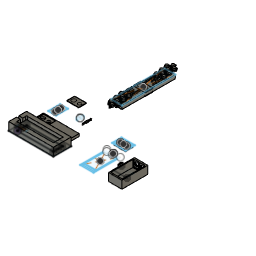
2020_09_27_9V Led 1W Experiments v4 (Autodesk Fusion 360 design; units mm, degrees)
Autodesk Fusion 360 part; units mm, degrees
sketch "Sketch1" plane through (0, 0, 0) normal (0, 0, 1) x (1, 0, 0)
  line L0 (0, 0) -> (80, 0)
  line L1 (80, 0) -> (80, 20)
  line L2 (80, 20) -> (0, 20)
  line L3 (0, 20) -> (0, 0)
  line L4 (-10, -10) -> (90, -10)
  line L5 (90, -10) -> (90, 30)
  line L6 (90, 30) -> (-10, 30)
  line L7 (-10, 30) -> (-10, -10)
  circle A0 centre (0, 20) radius 1.6
  circle A1 centre (80, 20) radius 1.6
  circle A2 centre (80, 0) radius 1.6
  circle A3 centre (0, 0) radius 1.6
  line L8 (-10, 12.5) -> (10, 12.5)
  line L9 (10, 12.5) -> (10, 7.5)
  line L10 (10, 7.5) -> (-10, 7.5)
  line L11 (-10, 7.5) -> (-10, 12.5)
  line L12 (-10, 12.5) -> (10, 7.5) construction
  line L13 (10, 12.5) -> (-10, 7.5) construction
  circle A4 centre (80, 10) radius 1.55
  line L14 (-1, -1) -> (81, -1)
  line L15 (81, -1) -> (81, 21)
  line L16 (81, 21) -> (-1, 21)
  line L17 (-1, 21) -> (-1, -1)
  point P0 (-10, 10)
  point P1 (0, 10)
  dimension "d1" = 80
  dimension "d2" = 20
  dimension "d3" = 10
  dimension "d10" = 3.2
  dimension "d12" = 5
  dimension "d18" = 3.1
  dimension "d21" = 1
  constraint horizontal L0
  constraint vertical L1
  constraint horizontal L2
  constraint vertical L3
  constraint coincident L0.start L3.end
  constraint coincident L2.end L3.start
  constraint coincident L1.end L2.start
  constraint coincident L0.end L1.start
  constraint equal A0 A1
  constraint equal A0 A3
  constraint equal A0 A2
  constraint midpoint L7 P0
  constraint horizontal L8
  constraint perpendicular L8 L9
  constraint parallel L8 L10
  constraint parallel L9 L11
  constraint coincident L12 P1
  constraint coincident L13 P1
  constraint midpoint L3 P1
  constraint midpoint L1 A4.centre
  measures "d1" distance of L0.start L0.end
  measures "d2" distance of L0.start L2.end
  measures "d10" diameter of A0
  measures "d12" distance of L8.end L9.end
  measures "d18" diameter of A4
extrude "Extrude1" add sketch "Sketch1" along normal blind 17.8 contours L4 L5 L6 L7 A0 A1 A2 A3 L8 L10 A4 L14 L15 L16 L17 makes body 1
extrude "Extrude3" add sketch "Sketch1" along normal blind 5.3 separate body contours L0 L3 A3 | L0 L3 A3 L14 L17 | L0 L1 L2 L3 A0 A1 A2 A3 L8 L9 L10 A4 | L0 A2 A3 L14 | L3 A3 L10 L17 | L0 L1 A2 | L0 L1 A2 L14 L15 | A3 L14 L17 | L3 L8 L10 L17 | L3 L8 L9 L10 | L1 A2 A4 L15 | A2 L14 L15 | L3 A0 L8 L17 | L1 A4 | L1 A4 L15 | L2 L3 A0 L16 L17 | L2 L3 A0 | L1 A1 A4 L15 | A4 L15 | A0 L16 L17 | L2 A0 A1 L16 | L1 L2 A1 | L1 L2 A1 L15 L16 | A1 L15 L16 makes body 2
move_body "Move1" bodies 2 to x (1, 0, 0) y (0, 1, 0) z (0, 0, 1) at (0, 0, 5.3)
extrude "Extrude4" add sketch "Sketch1" along normal blind 10.6 contours L0 L3 A3 | L0 L3 A3 L14 L17 | L0 L1 L2 L3 A0 A1 A2 A3 L8 L9 L10 A4 | L0 L1 A2 | L0 L1 A2 L14 L15 | A3 L14 L17 | A2 L14 L15 | L1 A4 | L1 A4 L15 | L2 L3 A0 L16 L17 | L2 L3 A0 | A4 L15 | A0 L16 L17 | L1 L2 A1 | L1 L2 A1 L15 L16 | A1 L15 L16 bodies 2 1
extrude "Extrude5" add sketch "Sketch1" along normal blind 5.5 separate body contours L0 L3 A3 | L0 L1 L2 L3 A0 A1 A2 A3 L8 L9 L10 A4 | L0 L1 A2 | L3 L8 L9 L10 | L1 A4 | L2 L3 A0 | L1 L2 A1 makes body 3
move_body "Move2" bodies 3 to x (1, 0, 0) y (0, 1, 0) z (0, 0, 1) at (0, 38, 0)
sketch "Sketch2" plane through (0, 0, 0) normal (1, 0, 0) x (0, 1, 0)
sketch "SquareBattery" plane through (0, 0, 0) normal (0, 0, 1) x (1, 0, 0)
  circle A0 centre (4.7694, 92.4101) radius 3.5
  circle A1 centre (4.7694, 79.4101) radius 4.5
  line L0 (4.7694, 79.4101) -> (4.7694, 92.4101)
  line L1 (13.5194, 99.1601) -> (-3.9806, 99.1601)
  line L2 (-3.9806, 99.1601) -> (-3.9806, 72.6601)
  line L3 (-3.9806, 72.6601) -> (13.5194, 72.6601)
  line L4 (13.5194, 72.6601) -> (13.5194, 99.1601)
  line L5 (13.5194, 99.1601) -> (-3.9806, 72.6601) construction
  line L6 (-3.9806, 99.1601) -> (13.5194, 72.6601) construction
  point P0 (4.7694, 85.9101)
  point P1 (4.7694, 85.9101)
  dimension "d25" = 7
  dimension "d26" = 9
  dimension "d27" = 13
  dimension "d28" = 17.5
  dimension "d29" = 26.5
  constraint coincident A1.centre L0.start
  constraint vertical L0
  constraint coincident A0.centre L0.end
  constraint midpoint L0 P1
  constraint horizontal L1
  constraint perpendicular L1 L2
  constraint parallel L1 L3
  constraint parallel L2 L4
  constraint coincident L5 P1
  constraint coincident L6 P1
  constraint coincident P1 P0
  measures "d25" diameter of A0
  measures "d26" diameter of A1
  measures "d27" distance of A1.centre A0.centre
  measures "d28" distance of L2.end L3.end
  measures "d29" distance of L1.end L2.end
extrude "Extrude6" add sketch "SquareBattery" against normal blind 3 separate body contours A0 | A1 makes body 4 at (8.0583, 91.2131, -2) makes body 5 at (9.247, 79.8582, -1)
extrude "Extrude7" add sketch "SquareBattery" along normal blind 1 contours A0 | A1 | L1 L2 L3 L4 bodies 4 5
move_body "Move3" bodies 4 to x (0, -1, 0) y (1, 0, 0) z (0, 0, 1) at (-58, 58, 0)
move_body "Move4" bodies 4 to x (1, 0, 0) y (0, 1, 0) z (0, 0, 1) at (-14.6601, -5.2306, 4.5)
move_body "Move5" bodies 4 to x (1, 0, 0) y (0, 1, 0) z (0, 0, 1) at (2, 0, 0)
copy_body "CopyPasteBodies1" bodies 4 makes body 6
move_body "Move6" bodies 6 to x (1, 0, 0) y (0, 1, 0) z (0, 0, 1) at (0, 69, 0)
combine "Combine1" operation cut target body 3 tool bodies 4
sketch "Zerodis6bz7yhokr1-02" plane through (0, 0, 0) normal (0, 0, 1) x (1, 0, 0)
  line L0 (41.1745, 98.5288) -> (49.3245, 98.5288)
  line L1 (49.3245, 98.5288) -> (49.3245, 91.2088)
  line L2 (49.3245, 91.2088) -> (41.1745, 91.2088)
  line L3 (41.1745, 91.2088) -> (41.1745, 98.5288)
  line L4 (45.2495, 98.5288) -> (45.2495, 91.2088) construction
  arc A0 (43.4578, 98.5288) -> (43.4578, 91.2088) centre (45.2495, 94.8688) ccw
  arc A1 (47.0411, 91.2088) -> (47.0411, 98.5288) centre (45.2495, 94.8688) ccw
  circle A2 centre (45.2495, 94.8688) radius 2.75
  line L5 (45.2495, 98.5288) -> (43.4578, 98.5288)
  line L6 (43.4578, 98.5288) -> (43.4578, 102.2288)
  line L7 (43.4578, 102.2288) -> (45.2495, 102.2288)
  line L8 (45.2495, 102.2288) -> (45.2495, 98.5288)
  line L9 (45.2495, 91.2088) -> (47.0411, 91.2088)
  line L10 (47.0411, 91.2088) -> (47.0411, 87.5088)
  line L11 (47.0411, 87.5088) -> (45.2495, 87.5088)
  line L12 (45.2495, 87.5088) -> (45.2495, 91.2088)
  line L13 (45.2495, 98.5288) -> (45.2495, 100.5288)
  line L14 (45.2495, 100.5288) -> (43.4578, 100.5288)
  line L15 (45.2495, 91.2088) -> (45.2495, 89.2088)
  line L16 (45.2495, 89.2088) -> (47.0411, 89.2088)
  line L17 (47.0411, 98.5288) -> (45.2495, 98.5288)
  line L18 (45.2495, 98.5288) -> (45.2495, 100.0288)
  line L19 (45.2495, 100.0288) -> (47.0411, 100.0288)
  line L20 (47.0411, 100.0288) -> (47.0411, 98.5288)
  line L21 (43.4578, 91.2088) -> (45.2495, 91.2088)
  line L22 (45.2495, 91.2088) -> (45.2495, 89.7088)
  line L23 (45.2495, 89.7088) -> (43.4578, 89.7088)
  line L24 (43.4578, 89.7088) -> (43.4578, 91.2088)
  dimension "d38" = 8.15
  dimension "d39" = 7.32
  dimension "d42" = 5.5
  dimension "d43" = 3.7
  dimension "d44" = 3.7
  dimension "d51" = 2
  dimension "d52" = 2
  dimension "d55" = 1.5
  dimension "d56" = 1.5
  constraint horizontal L0
  constraint vertical L1
  constraint horizontal L2
  constraint vertical L3
  constraint midpoint L0 L4.start
  constraint midpoint L2 L4.end
  constraint tangent L1 A0
  constraint coincident L0 A1.end
  constraint coincident L0 A0.start
  constraint coincident L2 A0.end
  constraint coincident L2 A1.start
  constraint concentric A0 A1
  constraint horizontal L5
  constraint vertical L6
  constraint horizontal L7
  constraint vertical L8
  constraint horizontal L9
  constraint vertical L10
  constraint horizontal L11
  constraint vertical L12
  constraint perpendicular L0 L13
  constraint coincident L6 L14.end
  constraint perpendicular L6 L14
  constraint perpendicular L2 L15
  constraint coincident L10 L16.end
  constraint perpendicular L10 L16
  constraint horizontal L17
  constraint vertical L18
  constraint horizontal L19
  constraint vertical L20
  constraint horizontal L21
  constraint vertical L22
  constraint horizontal L23
  constraint vertical L24
  measures "d38" distance of L0.start L0.end
  measures "d39" distance of L0.start L2.end
  measures "d42" diameter of A2
  measures "d43" distance of L4.start L7.end
  measures "d44" distance of L4.end L11.end
  measures "d51" distance of L4.start L13.end
  measures "d52" distance of L4.end L15.end
  measures "d55" distance of A1.end L19.end
  measures "d56" distance of A0.end L23.end
extrude "Extrude8" add sketch "Zerodis6bz7yhokr1-02" against normal blind 0.1 separate body contours L0 L5 L6 L8 L13 L14 L18 | L6 L7 L8 L14 | L2 L9 L10 L12 L15 L16 L22 | L10 L11 L12 L16 makes body 7 at (46.4439, 89.9755, 0) makes body 8 at (44.055, 100.9955, 0)
extrude "Extrude9" add sketch "Zerodis6bz7yhokr1-02" along normal blind 2.37 separate body contours L0 L2 A0 A1 L5 L9 L17 L21 | A2 makes body 9
extrude "Extrude10" add sketch "Zerodis6bz7yhokr1-02" along normal blind 5.1 contours A2 bodies 9
extrude "Extrude11" add sketch "Zerodis6bz7yhokr1-02" along normal blind 1.8 contours L0 L5 L6 L8 L13 L14 L18 | L2 L9 L10 L12 L15 L16 L22 bodies 7 8 9
extrude "Extrude12" add sketch "Zerodis6bz7yhokr1-02" along normal blind 1.8 contours L0 L8 L13 L17 L18 L19 L20 | L2 L12 L15 L21 L22 L23 L24 bodies 7
extrude "Extrude13" add sketch "Zerodis6bz7yhokr1-02" along normal blind 0.15 contours L6 L7 L8 L14 | L10 L11 L12 L16 bodies 7
copy_body "CopyPasteBodies2" bodies 7 makes body 10
move_body "Move7" bodies 10 to x (1, 0, 0) y (0, 1, 0) z (0, 0, 1) at (0, 200, 0)
copy_body "CopyPasteBodies3" bodies 10 makes body 11
move_body "Move8" bodies 11 to x (1, 0, 0) y (0, 1, 0) z (0, 0, 1) at (1.8025, -13.4584, 0)
copy_body "CopyPasteBodies4" bodies 11 makes body 12
move_body "Move9" bodies 12 to x (1, 0, 0) y (0, 1, 0) z (0, 0, 1) at (1.8025, -13.3382, 0)
copy_body "CopyPasteBodies5" bodies 10 12 11 makes body 13 makes body 14 makes body 15
move_body "Move10" bodies 13 14 15 to x (1, 0, 0) y (0, 1, 0) z (0, 0, 1) at (5.2658, 8.138, 0)
copy_body "CopyPasteBodies6" bodies 13 14 15 makes body 16 makes body 17 makes body 18
move_body "Move11" bodies 16 17 18 to x (1, 0, 0) y (0, 1, 0) z (0, 0, 1) at (7.5995, -5.0264, 0)
move_body "Move12" bodies 10 12 11 to x (1, 0, 0) y (0, 1, 0) z (0, 0, 1) at (-1, 0, 0)
sketch "Resistance" plane through (0, 0, 0) normal (0, 0, 1) x (1, 0, 0)
  line L0 (60.0185, 97.4679) -> (62.6185, 97.4679)
  line L1 (62.6185, 97.4679) -> (62.6185, 90.0679)
  line L2 (62.6185, 90.0679) -> (60.0185, 90.0679)
  line L3 (60.0185, 90.0679) -> (60.0185, 97.4679)
  line L4 (60.0185, 93.7679) -> (62.6185, 93.7679) construction
  line L5 (61.8685, 102.8813) -> (60.7685, 102.8813)
  line L6 (60.7685, 102.8813) -> (60.7685, 84.6546)
  line L7 (60.7685, 84.6546) -> (61.8685, 84.6546)
  line L8 (61.8685, 84.6546) -> (61.8685, 102.8813)
  line L9 (61.8685, 102.8813) -> (60.7685, 84.6546) construction
  line L10 (60.7685, 102.8813) -> (61.8685, 84.6546) construction
  circle A0 centre (61.3185, 84.6546) radius 1.25
  circle A1 centre (61.3185, 102.8813) radius 1.25
  point P0 (61.3185, 93.7679)
  dimension "d64" = 2.6
  dimension "d65" = 7.4
  dimension "d66" = 1.1
  dimension "d67" = 2.5
  dimension "d68" = 2.5
  constraint horizontal L0
  constraint vertical L1
  constraint horizontal L2
  constraint vertical L3
  constraint midpoint L3 L4.start
  constraint midpoint L1 L4.end
  constraint horizontal L5
  constraint perpendicular L5 L6
  constraint parallel L5 L7
  constraint parallel L6 L8
  constraint coincident L9 P0
  constraint coincident L10 P0
  constraint midpoint L4 P0
  constraint midpoint L7 A0.centre
  constraint midpoint L5 A1.centre
  measures "d64" distance of L0.start L0.end
  measures "d65" distance of L0.start L2.end
  measures "d66" distance of L6.end L7.end
  measures "d67" diameter of A0
  measures "d68" diameter of A1
extrude "Extrude14" add sketch "Resistance" along normal blind 2.5 separate body makes body 19
copy_body "CopyPasteBodies7" bodies 19 makes body 20
move_body "Move13" bodies 20 to x (1, 0, 0) y (0, 1, 0) z (0, 0, 1) at (1.3709, 160.9305, 0)
copy_body "CopyPasteBodies8" bodies 20 makes body 21
move_body "Move14" bodies 21 to x (1, 0, 0) y (0, 1, 0) z (0, 0, 1) at (-7.5014, 5.0154, 0)
copy_body "CopyPasteBodies9" bodies 21 makes body 22
move_body "Move15" bodies 22 to x (1, 0, 0) y (0, 1, 0) z (0, 0, 1) at (-6.3238, -7.9811, 0)
copy_body "CopyPasteBodies10" bodies 6 makes body 23
move_body "Move16" bodies 23 to x (1, 0, 0) y (0, 1, 0) z (0, 0, 1) at (39.8975, 108.9439, 0)
copy_body "CopyPasteBodies11" bodies 10 12 11 13 14 15 18 17 16 20 21 22 makes body 24 makes body 25 makes body 26 makes body 27 makes body 28 makes body 29 makes body 30 makes body 31 makes body 32 makes body 33 makes body 34 makes body 35
move_body "Move17" bodies 24 25 26 27 28 29 30 31 32 33 34 35 to x (-1, 0, 0) y (0, -1, 0) z (0, 0, 1) at (123.2951, 451.8879, 0)
move_body "Move18" bodies 26 35 32 28 27 24 25 33 34 29 30 31 to x (1, 0, 0) y (0, 1, 0) z (0, 0, 1) at (-15, 5, 0)
move_body "Move19" bodies 15 17 12 22 10 13 21 11 20 18 14 16 to x (1, 0, 0) y (0, 1, 0) z (0, 0, 1) at (0, -5, 0)
sketch "Sketch6" plane through (0, 0, 0) normal (0, 0, 1) x (1, 0, 0)
  line L0 (67.6833, 285.9439) -> (43.6833, 285.9439)
  line L1 (43.6833, 285.9439) -> (43.6833, 165.9439)
  line L2 (43.6833, 165.9439) -> (67.6833, 165.9439)
  line L3 (67.6833, 165.9439) -> (67.6833, 285.9439)
  line L4 (67.6833, 285.9439) -> (43.6833, 165.9439) construction
  line L5 (43.6833, 285.9439) -> (67.6833, 165.9439) construction
  point P0 (55.6833, 225.9439)
  dimension "d78" = 24
  dimension "d79" = 120
  constraint horizontal L0
  constraint perpendicular L0 L1
  constraint parallel L0 L2
  constraint parallel L1 L3
  constraint coincident L4 P0
  constraint coincident L5 P0
  measures "d78" distance of L1.end L2.end
  measures "d79" distance of L0.end L1.end
extrude "Extrude15" add sketch "Sketch6" against normal blind 8 separate body makes body 36
move_body "Move20" bodies 23 to x (1, 0, 0) y (0, 1, 0) z (0, 0, 1) at (0, 0, -5.5)
copy_body "CopyPasteBodies12" bodies 23 makes body 37
move_body "Move21" bodies 37 to x (-1, 0, 0) y (0, 1, 0) z (0, 0, -1) at (83.7951, 0, 0)
move_body "Move22" bodies 37 to x (1, 0, 0) y (0, 1, 0) z (0, 0, 1) at (26.5, 0, -8)
sketch "Sketch7" plane through (0, 0, 0) normal (0, 0, 1) x (1, 0, 0)
  line L0 (138.4181, 56.7453) -> (164.4181, 56.7453)
  line L1 (164.4181, 56.7453) -> (164.4181, 10.7453)
  line L2 (164.4181, 10.7453) -> (138.4181, 10.7453)
  line L3 (138.4181, 10.7453) -> (138.4181, 56.7453)
  line L4 (138.4181, 33.7453) -> (164.4181, 33.7453) construction
  line L5 (136.4181, 61.2453) -> (136.4181, 3.7453)
  line L6 (136.4181, 3.7453) -> (166.4181, 3.7453)
  line L7 (166.4181, 3.7453) -> (166.4181, 61.2453)
  line L8 (166.4181, 63.7453) -> (136.4181, 3.7453) construction
  line L9 (136.4181, 63.7453) -> (166.4181, 3.7453) construction
  line L10 (138.4181, 10.7453) -> (164.4181, 10.7453)
  line L11 (164.4181, 10.7453) -> (164.4181, 6.7453)
  line L12 (164.4181, 6.7453) -> (138.4181, 6.7453)
  line L13 (138.4181, 6.7453) -> (138.4181, 10.7453)
  line L14 (164.4181, 56.7453) -> (164.4181, 59.4453) construction
  line L15 (164.4181, 59.4453) -> (138.4181, 59.4453)
  line L16 (138.4181, 59.4453) -> (138.4181, 61.2453)
  line L17 (164.4181, 61.2453) -> (164.4181, 59.4453)
  line L18 (138.4181, 56.7453) -> (141.4181, 56.7453)
  line L19 (141.4181, 56.7453) -> (141.4181, 59.4453)
  line L20 (141.4181, 59.4453) -> (138.4181, 59.4453)
  line L21 (138.4181, 59.4453) -> (138.4181, 56.7453)
  line L22 (164.4181, 56.7453) -> (162.4181, 56.7453)
  line L23 (162.4181, 56.7453) -> (162.4181, 59.4453)
  line L24 (162.4181, 59.4453) -> (164.4181, 59.4453)
  line L25 (164.4181, 59.4453) -> (164.4181, 56.7453)
  line L26 (162.4181, 56.7453) -> (153.9181, 56.7453)
  line L27 (153.9181, 56.7453) -> (148.9181, 56.7453)
  line L28 (148.9181, 56.7453) -> (148.9181, 59.4453)
  line L29 (148.9181, 59.4453) -> (153.9181, 59.4453)
  line L30 (153.9181, 59.4453) -> (153.9181, 56.7453)
  line L31 (151.4181, 63.7453) -> (151.4181, 61.2453) construction
  line L32 (150.6681, 61.2453) -> (152.1681, 61.2453)
  line L33 (152.1681, 63.7453) -> (150.6681, 61.2453) construction
  line L34 (150.6681, 63.7453) -> (152.1681, 61.2453) construction
  line L35 (150.6681, 61.2453) -> (140.1681, 61.2453)
  line L36 (152.1681, 61.2453) -> (162.6681, 61.2453)
  line L37 (162.6681, 61.2453) -> (164.4181, 61.2453)
  line L38 (162.6681, 61.2453) -> (162.6681, 59.4453)
  line L39 (140.1681, 61.2453) -> (140.1681, 59.4453)
  line L40 (140.1681, 61.2453) -> (138.4181, 61.2453)
  line L41 (150.6681, 61.2453) -> (150.6681, 59.4453)
  line L42 (152.1681, 61.2453) -> (152.1681, 59.4453)
  line L43 (138.4181, 61.2453) -> (136.4181, 61.2453)
  line L44 (164.4181, 61.2453) -> (166.4181, 61.2453)
  point P0 (151.4181, 33.7453)
  point P1 (151.4181, 62.4953)
  dimension "d86" = 26
  dimension "d87" = 46
  dimension "d88" = 30
  dimension "d89" = 60
  dimension "d90" = 4
  dimension "d92" = 2.7
  dimension "d93" = 1.8
  dimension "d99" = 3
  dimension "d100" = 2
  dimension "d101" = 8.5
  dimension "d102" = 5
  dimension "d103" = 1.5
  dimension "d104" = 2.5
  dimension "d105" = 10.5
  dimension "d106" = 10.5
  dimension "d107" = 90
  constraint horizontal L0
  constraint vertical L1
  constraint horizontal L2
  constraint vertical L3
  constraint midpoint L3 L4.start
  constraint midpoint L1 L4.end
  constraint parallel L5 L7
  constraint coincident L8 P0
  constraint coincident L9 P0
  constraint midpoint L4 P0
  constraint horizontal L10
  constraint vertical L11
  constraint horizontal L12
  constraint vertical L13
  constraint perpendicular L0 L14
  constraint horizontal L15
  constraint vertical L16
  constraint vertical L17
  constraint horizontal L18
  constraint vertical L19
  constraint horizontal L20
  constraint vertical L21
  constraint horizontal L22
  constraint vertical L23
  constraint horizontal L24
  constraint vertical L25
  constraint perpendicular L23 L26
  constraint horizontal L27
  constraint vertical L28
  constraint horizontal L29
  constraint vertical L30
  constraint coincident L33 P1
  constraint coincident L34 P1
  constraint midpoint L31 P1
  constraint perpendicular L17 L37
  constraint coincident L24 L38.end
  constraint coincident L15 L38.end
  constraint vertical L39
  constraint perpendicular L16 L40
  constraint vertical L41
  constraint coincident L15 L41.end
  constraint coincident L29 L41.end
  constraint perpendicular L32 L42
  constraint perpendicular L5 L43
  constraint perpendicular L7 L44
  measures "d86" distance of L0.start L0.end
  measures "d87" distance of L0.start L2.end
  measures "d88" distance of L5.end L6.end
  measures "d89" distance of L9.start L5.end
  measures "d90" distance of L2.end L12.end
  measures "d92" distance of L0.end L14.end
  measures "d93" distance of L14.end L17.start
  measures "d99" distance of L0.start L18.end
  measures "d100" distance of L0.end L22.end
  measures "d101" distance of L22.end L26.end
  measures "d102" distance of L26.end L27.end
  measures "d103" distance of L32.start L32.end
  measures "d104" distance of L34.start L32.start
  measures "d105" distance of L32.start L35.end
  measures "d106" distance of L32.end L36.end
  measures "d107" angle of L37 L38
sketch "Sketch8" plane through (0, 0, 0) normal (0, 0, 1) x (1, 0, 0)
  line L0 (137.9586, 92.7983) -> (150.9586, 92.7983) construction
  circle A0 centre (150.9586, 92.7983) radius 5.25
  circle A1 centre (137.9586, 92.7983) radius 5.25
  circle A2 centre (137.9586, 92.7983) radius 4.5
  circle A3 centre (150.9586, 92.7983) radius 4.5
  line L1 (157.4586, 101.2983) -> (131.4586, 101.2983)
  line L2 (131.4586, 101.2983) -> (131.4586, 84.2983)
  line L3 (131.4586, 84.2983) -> (157.4586, 84.2983)
  line L4 (157.4586, 84.2983) -> (157.4586, 101.2983)
  line L5 (157.4586, 101.2983) -> (131.4586, 84.2983) construction
  line L6 (131.4586, 101.2983) -> (157.4586, 84.2983) construction
  line L7 (159.4586, 103.2983) -> (129.4586, 103.2983)
  line L8 (129.4586, 103.2983) -> (129.4586, 82.2983)
  line L9 (129.4586, 82.2983) -> (159.4586, 82.2983)
  line L10 (159.4586, 82.2983) -> (159.4586, 103.2983)
  point P0 (144.4586, 92.7983)
  dimension "d108" = 13
  dimension "d109" = 10.5
  dimension "d110" = 10.5
  dimension "d111" = 9
  dimension "d112" = 9
  dimension "d113" = 26
  dimension "d114" = 17
  dimension "d125" = 2
  constraint horizontal L0
  constraint coincident L0.end A0.centre
  constraint coincident L0.start A1.centre
  constraint concentric A1 A2
  constraint concentric A0 A3
  constraint horizontal L1
  constraint perpendicular L1 L2
  constraint parallel L1 L3
  constraint parallel L2 L4
  constraint coincident L5 P0
  constraint coincident L6 P0
  constraint midpoint L0 P0
  measures "d108" distance of L0.start L0.end
  measures "d109" diameter of A0
  measures "d110" diameter of A1
  measures "d111" diameter of A2
  measures "d112" diameter of A3
  measures "d113" distance of L2.end L3.end
  measures "d114" distance of L1.end L2.end
extrude "Extrude16" add sketch "Sketch8" against normal blind 3.5 separate body contours A0 | A1 | A2 | A3 | L1 L2 L3 L4 makes body 38
extrude "Extrude17" cut sketch "Sketch8" against normal blind 1.5 contours A0 | A1 bodies 38
extrude "Extrude18" cut sketch "Sketch8" against normal blind 3.5 contours A2 | A3 bodies 38
sketch "Sketch9" plane through (0, 0, -3.5) normal (0, 0, -1) x (1, 0, 0)
  circle A0 centre (150.9586, -92.7983) radius 4.5
  circle A1 centre (137.9586, -92.7983) radius 4.5
  line L0 (157.4586, -101.2983) -> (157.4586, -84.2983)
  line L1 (157.4586, -84.2983) -> (131.4586, -84.2983)
  line L2 (131.4586, -84.2983) -> (131.4586, -101.2983)
  line L3 (131.4586, -101.2983) -> (157.4586, -101.2983)
  line L4 (132.4586, -100.2983) -> (156.4586, -100.2983)
  line L5 (156.4586, -100.2983) -> (156.4586, -85.2983)
  line L6 (156.4586, -85.2983) -> (132.4586, -85.2983)
  line L7 (132.4586, -85.2983) -> (132.4586, -100.2983)
  line L8 (144.9586, -85.2983) -> (143.9586, -85.2983)
  line L9 (143.9586, -85.2983) -> (143.9586, -100.2983)
  line L10 (143.9586, -100.2983) -> (144.9586, -100.2983)
  line L11 (144.9586, -100.2983) -> (144.9586, -85.2983)
  line L12 (144.9586, -85.2983) -> (143.9586, -100.2983) construction
  line L13 (143.9586, -85.2983) -> (144.9586, -100.2983) construction
  point P0 (144.4586, -92.7983)
  point P1 (144.4586, -92.7983)
  dimension "d121" = -1
  dimension "d122" = 1
  constraint horizontal L8
  constraint perpendicular L8 L9
  constraint parallel L8 L10
  constraint parallel L9 L11
  constraint coincident L12 P1
  constraint coincident L13 P1
  constraint coincident P1 P0
  measures "d122" distance of L9.end L10.end
extrude "Extrude20" add sketch "Sketch8" against normal blind 55 contours L7 L8 L9 L10 bodies 38
extrude "Extrude19" add sketch "Sketch9" along normal blind 2 contours L0 L1 L2 L3 | L4 L6 L8 L9 L10 L11 bodies 38
sketch "Sketch10" plane through (0, 0, -55) normal (0, 0, -1) x (1, 0, 0)
  line L0 (157.4586, -84.2983) -> (157.4586, -101.2983)
  line L1 (157.4586, -101.2983) -> (131.4586, -101.2983)
  line L2 (131.4586, -101.2983) -> (131.4586, -84.2983)
  line L3 (131.4586, -84.2983) -> (157.4586, -84.2983)
  line L4 (159.4586, -103.2983) -> (159.4586, -82.2983)
  line L5 (159.4586, -82.2983) -> (129.4586, -82.2983)
  line L6 (129.4586, -82.2983) -> (129.4586, -103.2983)
  line L7 (129.4586, -103.2983) -> (159.4586, -103.2983)
  line L8 (129.4586, -103.2983) -> (129.4586, -85.7983)
  line L9 (129.4586, -85.7983) -> (159.4586, -85.7983)
  dimension "d130" = 17.5
  constraint coincident L6.end L7.start
  constraint perpendicular L7 L8
  constraint coincident L4 L9.end
  constraint perpendicular L4 L9
  measures "d130" distance of L6.end L8.end
extrude "Extrude21" add sketch "Sketch10" along normal blind 3 bodies 38
extrude "Extrude22" cut sketch "Sketch10" along normal blind 100 and the other way blind 100 contours L0 L2 L3 L4 L5 L6 L9 | L0 L2 L3 L9 bodies 38
move_body "Move23" bodies 38 to x (1, 0, 0) y (0, 0, -1) z (0, 1, 0) at (0, 82.2983, 82.2983)
move_body "Move24" bodies 38 to x (1, 0, 0) y (0, 1, 0) z (0, 0, 1) at (50, 0, 0)
named bodies: "HolderStick", "Stick", "SquareBattery", "SquareBattery (1)", "Zerodis6bz7yhokr1-02", "Zerodis6bz7yhokr1-02 (1)", "Zerodis6bz7yhokr1-02 (1) (1)", "Zerodis6bz7yhokr1-02 (1) (1) (1)", "Zerodis6bz7yhokr1-02 (1) (2)", "Zerodis6bz7yhokr1-02 (1) (1) (2)", "Zerodis6bz7yhokr1-02 (1) (1) (1) (1)", "Zerodis6bz7yhokr1-02 (1) (2) (1)", "Zerodis6bz7yhokr1-02 (1) (1) (2) (1)", "Zerodis6bz7yhokr1-02 (1) (1) (1) (1) (1)", "Resistance", "Resistance (1)", "Resistance (1) (1)", "Resistance (1) (1) (1)", "SquareBattery (1) (1)", "Zerodis6bz7yhokr1-02 (1) (3)", "Zerodis6bz7yhokr1-02 (1) (1) (1) (2)", "Zerodis6bz7yhokr1-02 (1) (1) (3)", "Zerodis6bz7yhokr1-02 (1) (2) (2)", "Zerodis6bz7yhokr1-02 (1) (1) (2) (2)", "Zerodis6bz7yhokr1-02 (1) (1) (2) (1) (1)", "Zerodis6bz7yhokr1-02 (1) (1) (1) (1) (1) (1)", "Zerodis6bz7yhokr1-02 (1) (2) (1) (1)", "Resistance (1) (2)", "Resistance (1) (1) (1) (1)", "Zerodis6bz7yhokr1-02 (1) (1) (1) (1) (1) (1) (1)", "Resistance (1) (1) (1) (1) (1)", "Kapla", "SquareBattery (1) (1) (1)", "BatteryMagnet"
